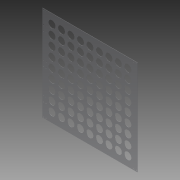
# Autodesk Inventor part: Plastic Funnel PIece
Saved by Autodesk Inventor 2014 (Build 180170000, 170)
## iProperties
Created: 2014-01-04
Part Number: Plastic Funnel PIece
Material: Polycarbonate, Clear
Document SubType Name: Modeling
Designer: Michael
Density: 1.2 g/cm^3
Appearance: Polycarbonate - Clear
Author: Michael
Autodesk Inventor part; units mm, degrees
ref_plane "YZ Plane" through (0, 0, 0) normal (1, 0, 0) x (0, 1, 0)
ref_plane "XZ Plane" through (0, 0, 0) normal (0, 1, 0) x (-1, 0, 0)
ref_plane "XY Plane" through (0, 0, 0) normal (0, 0, 1) x (1, 0, 0)
sketch "Sketch1" plane through (0, 0, 0) normal (0, 0, 1) x (1, 0, 0)
  line L0 (0, 0) -> (508, 0)
  line L1 (508, 0) -> (508, 508)
  line L2 (508, 508) -> (0, 508)
  line L3 (0, 508) -> (0, 0)
  circle A0 centre (6.35, 431.8) radius 2.4892
  line L4 (0, 254) -> (508, 254) construction
  circle A1 centre (6.35, 76.2) radius 2.4892
  line L5 (254, 508) -> (254, 0) construction
  line L6 (25.4, 482.6) -> (482.6, 482.6) construction
  line L7 (482.6, 482.6) -> (482.6, 25.4) construction
  line L8 (482.6, 25.4) -> (25.4, 25.4) construction
  line L9 (25.4, 25.4) -> (25.4, 482.6) construction
  circle A2 centre (19.05, 431.8) radius 2.4892
  circle A3 centre (19.05, 76.2) radius 2.4892
  circle A4 centre (6.35, 403.225) radius 2.4892
  circle A5 centre (19.05, 403.225) radius 2.4892
  circle A6 centre (6.35, 104.775) radius 2.4892
  circle A7 centre (19.05, 104.775) radius 2.4892
  circle A8 centre (6.35, 268.2875) radius 2.4892
  circle A9 centre (19.05, 268.2875) radius 2.4892
  circle A10 centre (6.35, 239.7125) radius 2.4892
  circle A11 centre (19.05, 239.7125) radius 2.4892
  line L10 (6.35, 431.8) -> (19.05, 431.8) construction
  circle A12 centre (6.35, 501.65) radius 2.4892
  circle A13 centre (19.05, 501.65) radius 2.4892
  circle A14 centre (501.65, 501.65) radius 2.4892
  circle A15 centre (488.95, 501.65) radius 2.4892
  circle A16 centre (488.95, 6.35) radius 2.4892
  circle A17 centre (501.65, 6.35) radius 2.4892
  circle A18 centre (19.05, 6.35) radius 2.4892
  circle A19 centre (6.35, 6.35) radius 2.4892
  dimension "d5" = 508
  dimension "d6" = 508
  dimension "d7" = 4.9784
  dimension "d9" = 6.35
  dimension "d12" = 25.4
  dimension "d41" = 4.9784
  dimension "d42" = 12.7
  dimension "d50" = 4.9784
  dimension "d51" = 4.9784
  dimension "d52" = 28.575
  dimension "d53" = 28.575
  dimension "d54" = 12.7
  dimension "d55" = 6.35
  dimension "d56" = 4.9784
  dimension "d59" = 12.7
  dimension "d62" = 28.575
  dimension "d65" = 6.35
  dimension "d66" = 76.2
  dimension "d67" = 4.9784
  dimension "d68" = 4.9784
  dimension "d69" = 6.35
  dimension "d70" = 6.35
  dimension "d71" = 12.7
  dimension "d72" = 6.35
  constraints: 22 end point, 20 centre point, 10 symmetric about line, 4 midpoint, 4 parallel, 3 horizontal, 2 perpendicular, 1 vertical, 20 other
  measures "d5" distance of L2.end L1.end
  measures "d6" distance of L1.end L0.end
  measures "d7" diameter of A0
  measures "d9" distance from line of L3 L10.start
  measures "d12" distance between parallel lines of L6 L2
  measures "d41" diameter of A2
  measures "d42" distance of L10.start L10.end
  measures "d50" diameter of A4
  measures "d51" diameter of A5
  measures "d52" distance of L10.start A4.centre
  measures "d53" distance of L10.end A5.centre
  measures "d54" distance of A5.centre A4.centre
  measures "d55" distance from line of L3 A4.centre
  measures "d56" diameter of A8
  measures "d59" distance of A8.centre A9.centre
  measures "d62" distance of A8.centre A10.centre
  measures "d65" distance from line of L3 A8.centre
  measures "d66" distance from line of L2 L10.start
  measures "d67" diameter of A12
  measures "d68" diameter of A13
  measures "d69" distance from line of L2 A12.centre
  measures "d70" distance from line of L3 A12.centre
  measures "d71" distance of A13.centre A12.centre
  measures "d72" distance from line of L2 A13.centre
extrude "Extrusion1" add sketch "Sketch1" along normal blind 1.5875
sketch "Sketch3" plane through (0, 0, 0) normal (0, 0, -1) x (-1, 0, 0)
  line L0 (-508, 508) -> (0, 508) projected
  line L1 (-508, 0) -> (-508, 508) projected
  circle A0 centre (-457.2, 457.2) radius 19.05
  dimension "d26" = 38.1
  dimension "d27" = 50.8
  dimension "d28" = 50.8
  constraints: 1 centre point
  measures "d26" diameter of A0
  measures "d27" distance from line of L0 A0.centre
  measures "d28" distance from line of L1 A0.centre
extrude "Extrusion3" cut sketch "Sketch3" against normal blind 1.5875
pattern_linear "Rectangular Pattern1" count 9 spacing 50.8 along (-1, 0, 0) count 9 spacing 50.8 along (0, -1, 0) of "Extrusion3"
equation "\"d9\" = d8"
equation "\"d53\" = d52"
equation "\"d72\" = d69"
equation "\"d8\" = 6.35"
body "Solid2"
